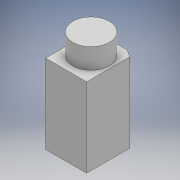
# Autodesk Inventor part: jack
Saved by Autodesk Inventor 2018 (Build 220112000, 112)
## iProperties
Created: 2017-12-11
Part Number: jack
Material: Generic
Document SubType Name: Modeling
Designer: ragna
Density: 1 g/cm^3
Appearance: Default
Author: ragna
Autodesk Inventor part; units mm, degrees
ref_plane "YZ Plane" through (0, 0, 0) normal (1, 0, 0) x (0, 1, 0)
ref_plane "XZ Plane" through (0, 0, 0) normal (0, 1, 0) x (-1, 0, 0)
ref_plane "XY Plane" through (0, 0, 0) normal (0, 0, 1) x (1, 0, 0)
sketch "Sketch1" plane through (0, 0, 0) normal (0, 0, 1) x (1, 0, 0)
  line L0 (0, 0) -> (9, 0)
  line L1 (9, 0) -> (9, 10.5)
  line L2 (9, 10.5) -> (0, 10.5)
  line L3 (0, 10.5) -> (0, 0)
  dimension "d0" = 9
  dimension "d1" = 10.5
  constraints: 8 end point, 2 parallel, 1 horizontal, 1 perpendicular
  measures "d0" distance of L2.end L1.end
  measures "d1" distance of L1.end L0.end
extrude "Extrusion1" add sketch "Sketch1" along normal blind 17.4
sketch "Sketch2" plane through (0, 0, 17.4) normal (0, 0, 1) x (1, 0, 0)
  line L0 (9, 10.5) -> (0, 10.5) construction
  line L1 (4.5, 10.5) -> (4.5, 0) construction
  circle A0 centre (4.5, 5.5) radius 4
  point P0 (0, 0)
  dimension "d4" = 8
  dimension "d5" = 5
  constraints: 2 end point, 1 centre point, 1 midpoint, 1 point on line, 1 vertical
  measures "d4" diameter of A0
  measures "d5" distance from line of L0 A0.centre
extrude "Extrusion2" add sketch "Sketch2" along normal blind 4.5
sketch "Sketch3" plane through (0, 0, 17.4) normal (0, 0, 1) x (1, 0, 0)
  line L0 (9, 10.5) -> (0, 10.5) construction
  line L1 (4.5, 10.5) -> (4.5, 0) construction
  line L2 (0, 0) -> (9, 0) construction
  line L3 (1.6586, 10.5) -> (0, 9.5141)
  line L4 (0, 10.5) -> (0, 0) projected
  line L5 (0, 9.5141) -> (0, 10.5)
  line L6 (0, 10.5) -> (1.6586, 10.5)
  line L7 (7.3414, 10.5) -> (9, 9.5141)
  line L8 (9, 9.5141) -> (9, 10.5)
  line L9 (9, 10.5) -> (7.3414, 10.5)
  constraints: 14 end point, 3 point on line, 3 symmetric about line, 2 midpoint, 1 collinear
extrude "Extrusion3" cut sketch "Sketch3" against normal through all
body "Solid1"
